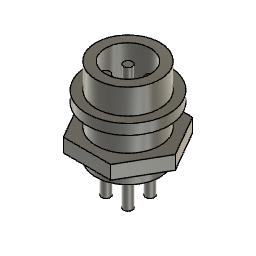
Device-LeakLevel-NodeController v5 (Autodesk Fusion 360 archive; units mm, degrees)
design "4pin round connector"
Autodesk Fusion 360 part; units mm, degrees
sketch "Sketch1" plane through (0, 0, 0) normal (0, 0, 1) x (1, 0, 0) in component "Socket"
  circle A0 centre (0, 0) radius 5.85
  circle A1 centre (2.0153, 2.0153) radius 0.8
  circle A2 centre (-2.0153, -2.0153) radius 0.8
  circle A3 centre (2.0153, -2.0153) radius 0.8
  circle A4 centre (-2.0153, 2.0153) radius 0.8
  circle A5 centre (0, 0) radius 7.5
  circle A6 centre (0, 0) radius 4.1
  line L0 (4.3301, -7.5) -> (8.6603, 0)
  line L1 (8.6603, 0) -> (4.3301, 7.5)
  line L2 (4.3301, 7.5) -> (-4.3301, 7.5)
  line L3 (-4.3301, 7.5) -> (-8.6603, 0)
  line L4 (-8.6603, 0) -> (-4.3301, -7.5)
  line L5 (-4.3301, -7.5) -> (4.3301, -7.5)
  arc A7 (0.7964, -4.0219) -> (-0.7959, -4.022) centre (0.0003, -4.1) ccw
  dimension "d2" = 1.6
  dimension "d4" = 1.6
  dimension "d11" = -1.75
  dimension "d23" = 1.6
  constraint coincident A0.centre A5.centre
  constraint concentric A0 A5
  measures "d2" diameter of A1
  measures "d4" diameter of A3
  measures "d23" diameter of A7
extrude "Extrude1" add sketch "Sketch1" along normal blind 1.9 contours A5 makes body 1 in component "Socket"
extrude "Extrude2" add sketch "Sketch1" along normal blind 6.5 contours A0 bodies 1 in component "Socket"
extrude "Extrude3" add sketch "Sketch1" along normal blind 4 separate body contours A1 | A2 | A3 | A4 makes body 2 at (2.8143, -2.0551, 2.6667) makes body 3 at (-1.2162, 1.9754, 2.6667) makes body 4 at (2.8143, 1.9754, 2.6667) makes body 5 at (-1.2162, -2.0551, 2.6667) in component "Socket"
extrude "Extrude4" add sketch "Sketch1" against normal blind 9 contours A0 | A6 A7 | A6 A7 bodies 1 2 3 4 5 in component "Socket"
extrude "Extrude5" add sketch "Sketch1" against normal blind 14.75 separate body contours A1 | A2 | A3 | A4 makes body 6 at (2.8143, -2.0551, -9.8333) makes body 7 at (-1.2162, 1.9754, -9.8333) makes body 8 at (-1.2162, -2.0551, -9.8333) makes body 9 at (2.8143, 1.9754, -9.8333) in component "Socket"
extrude "Extrude6" add sketch "Sketch1" 1 faces at (6.9003, -0.6632, 0) against normal blind 2.5 from surface at -4 separate body contours A5 L0 L1 | A5 L1 L2 | A5 L0 L5 | A5 L2 L3 | A5 L4 L5 | A5 L3 L4 on bodies 1 makes body 10 in component "Socket"
extrude "Extrude1'" add sketch "Sketch1" along normal up to surface (6.5 mm away) separate body contours A6 A7 picked at (0.0002, -3.8275) makes body 11
component "Socket" placed x (1, 0, 0) y (0, 1, 0) z (0, 0, 1) at (0, 0, 0)
equation "d17 = -9.00 mm + -5.75 mm"
equation "d23 = d2"
